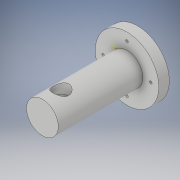
# Autodesk Inventor part: CrankP1_SBail
Saved by Autodesk Inventor 2019 (Build 230136000, 136)
## iProperties
Created: 2019-05-02
Part Number: CrankP1_SBail
Material: Generic
Document SubType Name: Modeling
Designer: samson.bailor
Density: 1 g/cm^3
Appearance: Default
Author: samson.bailor
Autodesk Inventor part; units mm, degrees
ref_plane "YZ Plane" through (0, 0, 0) normal (1, 0, 0) x (0, 1, 0)
ref_plane "XZ Plane" through (0, 0, 0) normal (0, 1, 0) x (-1, 0, 0)
ref_plane "Work Plane6" through (0, 0, 31.75) normal (0, 0, 1) x (1, 0, 0)
sketch "Sketch4" plane through (0, 0, 31.75) normal (0, 0, 1) x (1, 0, 0)
  line L0 (17.1377, 8.1273) -> (-8.2623, 8.1273) projected
  line L1 (4.4377, 8.1273) -> (4.4377, -17.2727)
  line L2 (-8.2623, -17.2727) -> (17.1377, -17.2727) projected
  circle A0 centre (4.4377, -4.5727) radius 25.4
  point P0 (0, 0)
  dimension "d11" = 50.8
  constraints: 3 midpoint, 2 end point, 1 centre point
  measures "d11" diameter of A0
extrude "Extrusion4" add sketch "Sketch4" along normal blind 101.6
ref_plane "Work Plane2" through (-8.2623, 8.1273, 0) normal (0, 1, 0) x (1, 0, 0)
sketch "Sketch5" plane through (-8.2623, 8.1273, 0) normal (0, 1, 0) x (1, 0, 0)
  line L0 (25.4, 0) -> (0, 0) projected
  line L1 (-12.7, -133.35) -> (38.1, -133.35) projected
  circle A0 centre (12.7, -111.125) radius 9.525
  point P0 (8.2623, 0)
  constraints: 1 centre point
extrude "Extrusion5" cut sketch "Sketch5" along normal blind 101.6
sketch "Sketch6" plane through (4.4377, 8.1273, 111.125) normal (0, 1, 0) x (1, 0, 0)
  circle A0 centre (0, 0) radius 9.525
  point P0 (-4.4377, 111.125)
  constraints: 1 centre point
extrude "Extrusion6" cut sketch "Sketch6" against normal blind 6.35
sketch "Sketch13" plane through (4.4377, -4.5727, 31.75) normal (0, 0, -1) x (-1, 0, 0)
  circle A0 centre (0, 0) radius 38.1
  point P0 (4.4377, 4.5727)
  dimension "d36" = 76.2
  constraints: 1 centre point
  measures "d36" diameter of A0
extrude "Extrusion11" add sketch "Sketch13" along normal blind 12.7
sketch "Sketch14" plane through (4.4377, -4.5727, 133.35) normal (0, 0, 1) x (1, 0, 0)
  circle A0 centre (0, 0) radius 19.05
  circle A1 centre (0, 0) radius 25.4
  point P0 (-4.4377, 4.5727)
  dimension "d39" = 38.1
  constraints: 2 centre point, 1 coincident
  measures "d39" diameter of A0
extrude "Extrusion12" cut sketch "Sketch14" against normal blind 101.6
sketch "Sketch15" plane through (4.4377, -4.5727, 31.75) normal (0, 0, 1) x (1, 0, 0)
  circle A0 centre (0, 0) radius 19.05 projected
  line L0 (-19.05, 0) -> (-38.1, 0)
  circle A1 centre (0, 0) radius 38.1 projected
  line L1 (0, 38.1) -> (0, 19.0375)
  line L2 (19.05, 0) -> (38.1, 0)
  line L3 (0, -19.05) -> (0, -38.1)
  circle A2 centre (-28.575, 0) radius 1.5875
  circle A3 centre (28.575, 0) radius 1.5875
  circle A4 centre (0, 28.5687) radius 1.5875
  circle A5 centre (0, -28.575) radius 1.5875
  point P0 (-4.4377, 4.5727)
  dimension "d42" = 3.175
  dimension "d43" = 3.175
  dimension "d44" = 3.175
  dimension "d45" = 3.175
  constraints: 8 end point, 7 point on circle, 4 centre point, 4 midpoint, 2 horizontal, 1 perpendicular, 1 vertical
  measures "d42" diameter of A2
  measures "d43" diameter of A3
  measures "d44" diameter of A4
  measures "d45" diameter of A5
extrude "Extrusion13" cut sketch "Sketch15" against normal blind 101.6 contours A2 L0 | L0 A2 | A5 L3 | L3 A5 | A4 L1 | L1 A4 | A3 L2 | L2 A3
body "Solid1"
